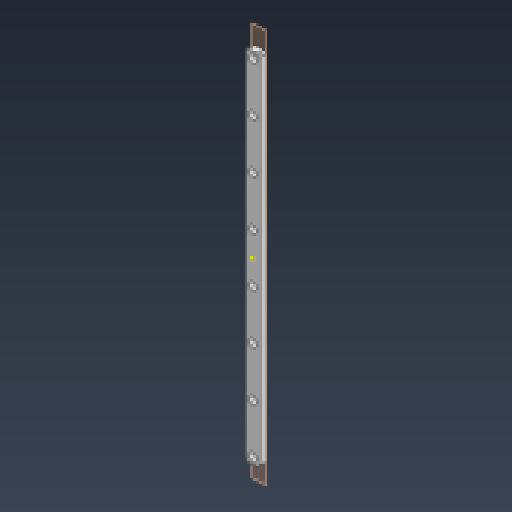
# Autodesk Inventor part: petg_holder_2
Saved by Autodesk Inventor 2023 (Build 270158000, 158)
## iProperties
Created: 2026-01-24
Part Number: petg_holder_2
Material: Generic
Document SubType Name: Modeling
Designer: szymo
Density: 1 g/cm^3
Appearance: Default
Author: szymo
Autodesk Inventor part; units mm, degrees
ref_plane "YZ Plane" through (0, 0, 0) normal (1, 0, 0) x (0, 1, 0)
ref_plane "XZ Plane" through (0, 0, 0) normal (0, 1, 0) x (-1, 0, 0)
ref_plane "XY Plane" through (0, 0, 0) normal (0, 0, 1) x (1, 0, 0)
ref_plane "Work Plane1" through (0, 0, 0) normal (0, 0, 1) x (1, 0, 0)
sketch "Sketch1" plane through (0, 0, 0) normal (0, 0, 1) x (1, 0, 0)
  circle A0 centre (0, 80) radius 1.8 projected
  circle A1 centre (0, 11.4286) radius 1.8 projected
  circle A2 centre (0, -34.2857) radius 1.8 projected
  circle A3 centre (0, -80) radius 1.8 projected
  circle A4 centre (0, -57.1429) radius 1.8 projected
  circle A5 centre (0, -11.4286) radius 1.8 projected
  circle A6 centre (0, 57.1429) radius 1.8 projected
  circle A7 centre (0, 34.2857) radius 1.8 projected
  line L0 (-3, 83) -> (3, 83) projected
  line L1 (-3, -83) -> (-3, 83) projected
  line L2 (3, -83) -> (-3, -83) projected
  line L3 (3, -83) -> (3, 83) projected
  point P0 (0, 0)
extrude "Extrusion1" add sketch "Sketch1" along normal blind 3
sketch "Sketch2" plane through (0, 0, 3) normal (0, 0, 1) x (1, 0, 0)
  point P0 (0, 0)
fillet "Fillet1" radius 1 4 edges at (3, 83, 1.5) (-3, 83, 1.5) (-3, -83, 1.5) (3, -83, 1.5)
body "Solid1"
